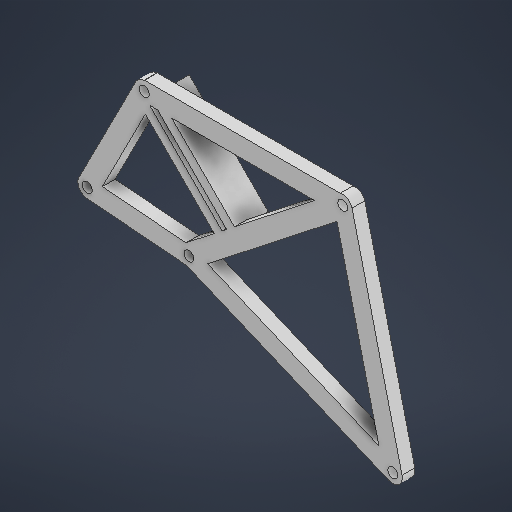
# Autodesk Inventor part: Part379
Saved by Autodesk Inventor 2025 (Build 290162000, 162)
## iProperties
Created: 2024-07-16
Part Number: Part379
Material: Generic
Document SubType Name: Modeling
Designer: Windows 7 was better
Density: 1 g/cm^3
Appearance: Default
Author: Windows 7 was better
Autodesk Inventor part; units mm, degrees
ref_plane "YZ Plane" through (0, 0, 0) normal (1, 0, 0) x (0, 1, 0)
ref_plane "XZ Plane" through (0, 0, 0) normal (0, 1, 0) x (-1, 0, 0)
ref_plane "XY Plane" through (0, 0, 0) normal (0, 0, 1) x (1, 0, 0)
sketch "Sketch1" plane through (0, 0, 0) normal (0, 0, 1) x (1, 0, 0)
  circle A0 centre (54.9228, 20.0746) radius 1.5 projected
  circle A1 centre (117.0828, 20.2746) radius 1.5 projected
  circle A2 centre (68.8728, -17.5454) radius 1.5 projected
  circle A3 centre (37.0628, -14.9054) radius 1.5 projected
  circle A4 centre (132.7528, -44.3954) radius 1.5 projected
  line L0 (54.9228, 20.0746) -> (117.0828, 20.2746) construction
  line L1 (117.0828, 20.2746) -> (132.7528, -44.3954) construction
  line L2 (132.7528, -44.3954) -> (68.8728, -17.5454) construction
  line L3 (68.8728, -17.5454) -> (37.0628, -14.9054) construction
  line L4 (37.0628, -14.9054) -> (54.9228, 20.0746) construction
  line L5 (68.8728, -17.5454) -> (117.0828, 20.2746) construction
  line L6 (117.0828, 23.1746) -> (54.9228, 23.1746)
  line L7 (54.9228, 23.1746) -> (54.9228, 17.1746)
  line L8 (54.9228, 17.1746) -> (117.0828, 17.1746)
  line L9 (117.0828, 17.1746) -> (117.0828, 23.1746)
  line L10 (117.0828, 23.1746) -> (54.9228, 17.1746) construction
  line L11 (54.9228, 23.1746) -> (117.0828, 17.1746) construction
  line L12 (34.3909, -13.5412) -> (52.2509, 21.4388)
  line L13 (52.2509, 21.4388) -> (57.5946, 18.7104)
  line L14 (57.5946, 18.7104) -> (39.7346, -16.2696)
  line L15 (39.7346, -16.2696) -> (34.3909, -13.5412)
  line L16 (34.3909, -13.5412) -> (57.5946, 18.7104) construction
  line L17 (52.2509, 21.4388) -> (39.7346, -16.2696) construction
  line L18 (37.3109, -11.9157) -> (69.1209, -14.5557)
  line L19 (69.1209, -14.5557) -> (68.6246, -20.5351)
  line L20 (68.6246, -20.5351) -> (36.8146, -17.8951)
  line L21 (36.8146, -17.8951) -> (37.3109, -11.9157)
  line L22 (37.3109, -11.9157) -> (68.6246, -20.5351) construction
  line L23 (69.1209, -14.5557) -> (36.8146, -17.8951) construction
  line L24 (67.0211, -15.185) -> (115.2311, 22.635)
  line L25 (115.2311, 22.635) -> (118.9344, 17.9142)
  line L26 (118.9344, 17.9142) -> (70.7244, -19.9058)
  line L27 (70.7244, -19.9058) -> (67.0211, -15.185)
  line L28 (67.0211, -15.185) -> (118.9344, 17.9142) construction
  line L29 (115.2311, 22.635) -> (70.7244, -19.9058) construction
  line L30 (70.0352, -14.7798) -> (133.9152, -41.6298)
  line L31 (133.9152, -41.6298) -> (131.5903, -47.161)
  line L32 (131.5903, -47.161) -> (67.7103, -20.311)
  line L33 (67.7103, -20.311) -> (70.0352, -14.7798)
  line L34 (70.0352, -14.7798) -> (131.5903, -47.161) construction
  line L35 (133.9152, -41.6298) -> (67.7103, -20.311) construction
  line L36 (114.1671, 19.5681) -> (129.8371, -45.1019)
  line L37 (129.8371, -45.1019) -> (135.6684, -43.6889)
  line L38 (135.6684, -43.6889) -> (119.9984, 20.9811)
  line L39 (119.9984, 20.9811) -> (114.1671, 19.5681)
  line L40 (114.1671, 19.5681) -> (135.6684, -43.6889) construction
  line L41 (129.8371, -45.1019) -> (119.9984, 20.9811) construction
  circle A5 centre (68.8728, -17.5454) radius 3
  circle A6 centre (132.7528, -44.3954) radius 3
  circle A7 centre (37.0628, -14.9054) radius 3
  circle A8 centre (54.9228, 20.0746) radius 3
  circle A9 centre (117.0828, 20.2746) radius 3
  circle A10 centre (54.9228, 20.0746) radius 1.55
  circle A11 centre (117.0828, 20.2746) radius 1.55
  circle A12 centre (132.7528, -44.3954) radius 1.55
  circle A13 centre (68.8728, -17.5454) radius 1.55
  circle A14 centre (37.0628, -14.9054) radius 1.55
  point P0 (0, 0)
  point P1 (86.0028, 20.1746)
  point P2 (45.9928, 2.5846)
  point P3 (52.9678, -16.2254)
  point P4 (92.9778, 1.3646)
  point P5 (100.8128, -30.9704)
  point P6 (124.9178, -12.0604)
  point P7 (67.9475, -14.4583)
  point P8 (41.7688, -12.2857)
  point P9 (56.8105, 17.1746)
  point P10 (108.2706, 17.1746)
  point P11 (74.7386, -16.7567)
  point P12 (115.2653, 15.0359)
  point P13 (128.438, -39.3276)
  point P14 (68.1497, -20.4957)
  point P15 (116.3146, 23.1746)
  point P16 (54.9228, 23.0746)
  dimension "d0" = 6
  dimension "d1" = 6
  dimension "d2" = 6
  dimension "d3" = 6
  dimension "d4" = 6
  dimension "d5" = 6
  dimension "d6" = 6
  dimension "d7" = 6
  dimension "d8" = 6
  dimension "d9" = 6
  dimension "d10" = 6
  dimension "d28" = 3.1
  dimension "d29" = 3.1
  dimension "d30" = 3.1
  dimension "d31" = 3.1
  dimension "d32" = 3.1
  constraints: 84 end point, 18 midpoint, 17 parallel, 10 centre point, 10 coincident, 6 perpendicular, 1 horizontal
  measures "d0" distance of L7.end L6.end
  measures "d1" distance of L12.end L13.end
  measures "d2" distance of L18.end L19.end
  measures "d3" distance of L24.end L25.end
  measures "d4" distance of L30.end L31.end
  measures "d5" distance of L37.end L36.end
  measures "d6" diameter of A5
  measures "d7" diameter of A6
  measures "d8" diameter of A7
  measures "d9" diameter of A8
  measures "d10" diameter of A9
  measures "d28" diameter of A10
  measures "d29" diameter of A11
  measures "d30" diameter of A12
  measures "d31" diameter of A13
  measures "d32" diameter of A14
extrude "Extrusion1" add sketch "Sketch1" along normal blind 4 contours A0 L7 A10 L13 | A0 L13 A10 L7 | L13 A10 L7 A0 | A0 L7 A10 L13 | A10 L13 A8 L7 | L7 A8 L13 A10 | L13 A8 L8 L7 A10 | A10 L7 L8 A8 L13 | L7 L6 A9 L24 L8 L14 A8 | L14 L8 A8 | A8 L8 L14 L18 A7 L12 | A7 L21 A14 L15 | L15 A14 L21 A7 | A9 L39 A11 L9 L6 | L6 L9 A11 L25 A9 | L24 A9 L36 L8 | L8 L36 L26 L30 A5 L18 L24 | L18 L24 A5 L32 L20 A7 L14 | L14 A7 L18 | A14 L21 A3 L15 | L15 A3 L21 A14 | A7 L15 A14 L21 | L21 A14 L15 A7 | A9 L25 A11 L39 | L38 A6 L30 L36 L26 A9 | L25 A11 L39 A9 | L36 A9 L9 L8 | L8 L9 A9 L26 L36 | L18 A5 L24 | A14 L15 A3 L21 | L21 A3 L15 A14 | L32 A5 L20 | L20 A5 L26 L30 L36 A6 L32 | A11 L39 A1 L9 | L9 A1 L25 A11 | A6 L31 A12 L37 | L37 A12 L31 A6 | A11 L25 A1 L39 | L25 A1 L39 A11 | L39 A11 L9 A9 | A5 L33 A13 L19 | L19 A13 L27 A5 | L27 A13 L33 A5 | A5 L33 A13 L19 | L19 A13 L27 A5 | A6 L37 A12 L31 | A12 L31 A4 L37 | L37 A4 L31 A12 | A6 L36 L30 | L31 A12 L37 A6 | A9 L9 A11 L25 | L39 A1 L9 A11 | L26 A5 L30 | A13 L33 A2 L19 | L19 A2 L27 A13 | A5 L27 A13 L33 | L27 A2 L33 A13 | A13 L33 A2 L19 | L19 A2 L27 A13 | A12 L37 A4 L31 | L31 A4 L37 A12 | A11 L9 A1 L25 | A13 L27 A2 L33
sketch "Sketch2" plane through (0, 0, 4) normal (0, 0, 1) x (1, 0, 0)
  circle A0 centre (117.0828, 20.2746) radius 1.5 construction
  circle A1 centre (68.8728, -17.5454) radius 1.5 construction
  line L0 (117.0828, 20.2746) -> (68.8728, -17.5454) construction
  circle A2 centre (54.9228, 20.0746) radius 1.5 construction
  line L1 (54.9228, 20.0746) -> (82.1371, -7.1397) construction
  line L2 (54.9228, 20.0746) -> (93.4096, 20.0746) construction
  line L3 (81.6114, -5.1998) -> (56.8627, 19.5489) construction
  line L4 (56.8627, 19.5489) -> (55.4485, 18.1347) construction
  line L5 (55.4485, 18.1347) -> (80.1972, -6.614) construction
  line L6 (80.1972, -6.614) -> (81.6114, -5.1998) construction
  line L7 (81.6114, -5.1998) -> (55.4485, 18.1347) construction
  line L8 (56.8627, 19.5489) -> (80.1972, -6.614) construction
  line L9 (56.8627, 19.5489) -> (81.6114, -5.1998)
  line L10 (81.6114, -5.1998) -> (83.7327, -3.0785)
  line L11 (83.7327, -3.0785) -> (58.984, 21.6702)
  line L12 (58.984, 21.6702) -> (56.8627, 19.5489)
  line L13 (80.1972, -6.614) -> (55.4485, 18.1347)
  line L14 (55.4485, 18.1347) -> (53.3271, 16.0134)
  line L15 (53.3271, 16.0134) -> (78.0759, -8.7354)
  line L16 (78.0759, -8.7354) -> (80.1972, -6.614)
  line L17 (80.1972, -6.614) -> (55.4485, 18.1347)
  line L18 (55.4485, 18.1347) -> (55.5192, 18.2054)
  line L19 (55.5192, 18.2054) -> (80.2679, -6.5433)
  line L20 (80.2679, -6.5433) -> (80.1972, -6.614)
  line L21 (81.6114, -5.1998) -> (56.8627, 19.5489)
  line L22 (56.8627, 19.5489) -> (56.792, 19.4782)
  line L23 (56.792, 19.4782) -> (81.5407, -5.2705)
  line L24 (81.5407, -5.2705) -> (81.6114, -5.1998)
  point P0 (0, 0)
  point P1 (68.5299, 6.4674)
  dimension "d13" = 45
  dimension "d14" = 35
  dimension "d15" = 2
  dimension "d16" = 3
  dimension "d17" = 3
  dimension "d33" = 0.1
  dimension "d34" = 0.1
  constraints: 50 end point, 12 equal length, 6 perpendicular, 3 midpoint, 1 horizontal, 1 point on line
  measures "d13" angle of L1 L2
  measures "d14" distance of L3.start L3.end
  measures "d15" distance of L4.end L3.end
  measures "d16" distance of L10.end L3.start
  measures "d17" distance of L14.end L4.end
  measures "d33" distance of L4.end L18.end
  measures "d34" distance of L22.end L3.end
extrude "Extrusion2" add sketch "Sketch2" against normal blind 10
fillet "Fillet1" radius 1 2 edges at (69.1663, 7.1038, -6) (67.8935, 5.831, -6)
sketch "Sketch3" plane through (0, 0, 4) normal (0, 0, 1) x (1, 0, 0)
  circle A0 centre (37.0628, -14.9054) radius 1.5 projected
  circle A1 centre (54.9228, 20.0746) radius 1.5 projected
  circle A2 centre (68.8728, -17.5454) radius 1.5 projected
  circle A3 centre (132.7528, -44.3954) radius 1.5 projected
  circle A4 centre (117.0828, 20.2746) radius 1.5 projected
  circle A5 centre (37.0628, -14.9054) radius 1.55
  circle A6 centre (68.8728, -17.5454) radius 1.55
  circle A7 centre (132.7528, -44.3954) radius 1.55
  circle A8 centre (117.0828, 20.2746) radius 1.55
  circle A9 centre (54.9228, 20.0746) radius 1.55
  point P0 (0, 0)
  dimension "d21" = 0.05
  dimension "d22" = 0.05
  dimension "d23" = 0.05
  dimension "d24" = 0.05
  dimension "d25" = 0.05
  constraints: 5 centre point
  measures "d21" radial gap between concentric circles of A0 A5
  measures "d22" radial gap between concentric circles of A2 A6
  measures "d23" radial gap between concentric circles of A3 A7
  measures "d24" radial gap between concentric circles of A4 A8
  measures "d25" radial gap between concentric circles of A1 A9
extrude "Extrusion3" cut sketch "Sketch3" against normal blind 4 contours A2 | A5 | A6 | A7 | A8 | A9
body "Solid1"
